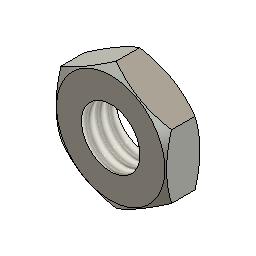
LumenPnp-Adj-Plate-Leg (Autodesk Fusion 360 archive; units mm, degrees)
design "Hexagon Nut BS 4183 - M5 Steel 6 Plain"
description: Hexagon Nut BS 4183 - M5
part number: HN BS 4183 - M5 Steel 6 Plain
Autodesk Fusion 360 part; units mm, degrees
sketch "Sketch1" plane through (0, 0, 0) normal (0, 1, 0) x (1, 0, 0)
  line L0 (0, 0) -> (0, -2.5)
  line L1 (-2.5, 0) -> (-3.92, 0)
  line L2 (-3.92, 0) -> (-4.62, -0.4041)
  line L3 (-4.62, -0.4041) -> (-4.62, -2.0959)
  line L4 (-4.62, -2.0959) -> (-3.92, -2.5)
  line L5 (-3.92, -2.5) -> (-2.5, -2.5)
  line L6 (-2.5, -2.5) -> (-2.5, 0)
  dimension "d121" = 5
  dimension "d122" = 30
  dimension "d123" = 30
  dimension "d125" = 7.84
  dimension "d128" = 9.24
  dimension "d153" = 2.5
  constraint vertical L0
  constraint coincident L0 L0.end
  constraint coincident origin L0
  constraint coincident L0.start L1
  constraint coincident L0.start origin
  constraint vertical L1.end L4.end
  constraint coincident L0.end L5
  constraint horizontal L1
  measures "d122" angle of L1 L2
  measures "d123" angle of L4 L5
  measures "d153" distance of L1 L5
revolve "Revolve1" add sketch "Sketch1" angle 360 about axis through (0, 0, 0) along (0, 0, 1)
sketch "Sketch8" plane through (0, 0, 2.5) normal (0, 0, 1) x (1, 0, 0)
  line L0 (-4, -2.3118) -> (-4, 2.3118)
  circle A0 centre (0, 0) radius 2.5
  circle A1 centre (0, 0) radius 4.62
  dimension "d114" = 4
  constraint coincident L0.end A1
  constraint coincident L0.start A1
  constraint vertical L0
  measures "d114" distance of A0.centre L0
extrude "Extrude5" cut sketch "Sketch8" against normal blind 2.5 contours L0 A1 picked at (-4.1, -0.5631)
pattern_circular "C-Pattern2" count 6 over 360 about axis through (0, 0, 1.75) along (0, 0, 1) of "Extrude5"
thread "Thread3" "ISO Metric profile 5.0 M5x0.8 M5x0.8 6H" major diameter 5.12 minor diameter 4.234 pitch 0.8 angle 60 resizes the face on face at (-2.4969, 0.1246, 1.6667)
equation "adsk_nheig = 2.50 mm"
equation "adsk_maxdia = 9.24 mm"
equation "adsk_nomdia = 5.00 mm"
equation "d89 = -adsk_nheig"
equation "adsk_waflat = 8.00 mm"
equation "d114 = adsk_waflat / 2"
equation "adsk_chamang1 = 30 deg"
equation "adsk_chamang2 = 30 deg"
equation "d121 = adsk_nomdia"
equation "d122 = adsk_chamang1"
equation "d123 = adsk_chamang2"
equation "d125 = adsk_beardia"
equation "d128 = adsk_maxdia"
equation "d147 = adsk_nheig"
equation "adsk_beardia = adsk_waflat * 0.98"
equation "d153 = adsk_nheig"

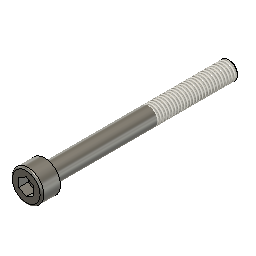
design "Hexagon Socket Head Cap Screw DIN EN ISO 4762 - M5 x 50 Steel 4.6 Plain"
description: Hexagon Socket Head Cap Screw DIN EN ISO 4762 - M5 x 50
part number: DIN EN ISO 4762 - M5 x 50 Steel 4.6 Plain
Autodesk Fusion 360 part; units mm, degrees
sketch "Sketch1" plane through (0, 0, 0) normal (0, 1, 0) x (1, 0, 0)
  line L0 (-2.5, 0) -> (-2.5, 50)
  line L1 (-2.5, 50) -> (0, 50)
  line L2 (0, 50) -> (0, -5)
  line L3 (-2.5, 0) -> (-4.25, 0)
  line L4 (-4.25, 0) -> (-4.25, -5)
  line L5 (-4.25, -5) -> (0, -5)
  dimension "d9" = 5
  dimension "d106" = 5
  dimension "d107" = 50
  dimension "d116" = 8.5
  constraint perpendicular L0 L1
  constraint collinear origin L1.end L2.end
  constraint perpendicular L0 L3
  constraint coincident origin L3
  constraint vertical L2
  constraint coincident L2 L5.end
  constraint perpendicular L2 L5
  measures "d106" distance of L3 L5
  measures "d107" distance of origin L1
revolve "Revolve1" add sketch "Sketch1" angle 360 about axis through (0, 0, -50) along (0, 0, 1)
ref_plane "WorkPlane1" through (0, 0, 5) normal (0, 0, 1) x (1, 0, 0)
sketch "Sketch6" plane through (0, 0, 5) normal (0, 0, 1) x (1, 0, 0)
  line L0 (-2, 1.1547) -> (-2, -1.1547)
  line L1 (-2, -1.1547) -> (0, -2.3094)
  line L2 (0, -2.3094) -> (2, -1.1547)
  line L3 (2, -1.1547) -> (2, 1.1547)
  line L4 (2, 1.1547) -> (0, 2.3094)
  line L5 (0, 2.3094) -> (-2, 1.1547)
  dimension "d117" = 4
  constraint vertical L0
  measures "d117" distance of L0 L3
extrude "Extrude1" cut sketch "Sketch6" against normal blind 2.5
extrude "Extrude2" cut 1 faces at (0.6667, -0.3849, 2.5) along direction (0, 0, -1) blind 2.5 draft -85
fillet "Fillet4" radius 0.5 1 edges at (-3.9624, 1.5369, 5)
thread "Thread3" "ISO Metric profile 5.0 M5x0.8 M5x0.8 6g" major diameter 4.901 minor diameter 3.9895 pitch 0.8 angle 60 resizes the face on face at (-2.4876, 0.2489, -33.3333) from (0, 0, -28) to (0, 0, -50)
sketch "Sketch7" plane through (0, 0, 0) normal (0, 1, 0) x (1, 0, 0)
  line L0 (-2.55, 50) -> (-2.55, 49.5)
  line L1 (-2.55, 49.5) -> (-2.05, 50)
  line L2 (0, 50) -> (0, -5)
  line L3 (-2.55, 50) -> (0, 50)
  dimension "d101" = 45
  dimension "d112" = 0.5
  dimension "d113" = 2.55
  constraint coincident L2.start L3.end
  constraint perpendicular L2 L3
  constraint coincident L1.end L3
  constraint perpendicular L0 L3
  measures "d101" angle of L0 L1
  measures "d112" distance of L0.end L3
  measures "d113" distance of L0 L2.start
revolve "Revolve3" cut sketch "Sketch7" angle 360 about axis through (0, 0, 1.75) along (0, 0, 1)
equation "d9 = adsk_nomdia"
equation "adsk_nomlen = 50.00 mm"
equation "adsk_headh = 5.00 mm"
equation "adsk_headdia = 8.50 mm"
equation "adsk_nomdia = 5.00 mm"
equation "adsk_philwidth = 4.00 mm"
equation "d31 = -adsk_phildepth"
equation "adsk_phildepth = 2.50 mm"
equation "d71 = adsk_headh"
equation "d76 = -adsk_phildepth"
equation "adsk_thrlen = 22.00 mm"
equation "d86 = adsk_nomdia * 0.1"
equation "adsk_startang = 45.00 deg"
equation "d101 = adsk_startang"
equation "adsk_pitch1 = 0.80 mm"
equation "adsk_startlen = 0.50 mm"
equation "d106 = adsk_headh"
equation "d107 = adsk_nomlen"
equation "d112 = adsk_startlen"
equation "d113 = adsk_nomdia * 0.51"
equation "d115 = min(adsk_thrlen; adsk_nomlen - 0.001 mm)"
equation "d116 = adsk_headdia"
equation "d117 = adsk_philwidth"
